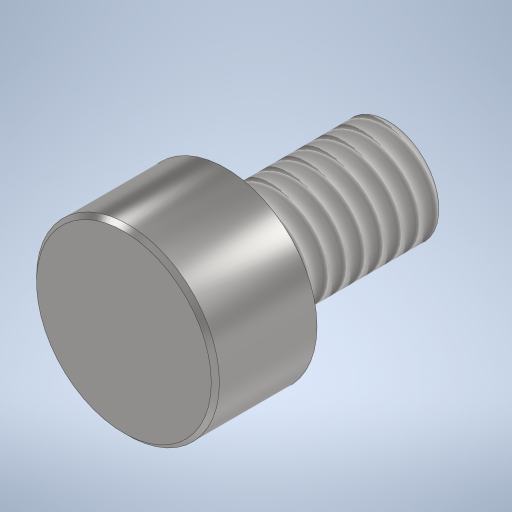
# Autodesk Inventor part: M2.5×4
Saved by Autodesk Inventor 2024 (Build 280153000, 153)
## iProperties
Created: 2025-03-04
Part Number: M2.5×4
Material: ステンレス鋼
Document SubType Name: Modeling
Designer: 1412z
Density: 8 g/cm^3
Appearance: 半つや出し
Author: 1412z
Autodesk Inventor part; units mm, degrees
ref_plane "YZ Plane" through (0, 0, 0) normal (1, 0, 0) x (0, 1, 0)
ref_plane "XZ Plane" through (0, 0, 0) normal (0, 1, 0) x (-1, 0, 0)
ref_plane "XY Plane" through (0, 0, 0) normal (0, 0, 1) x (1, 0, 0)
sketch "スケッチ1" plane through (0, 0, 0) normal (0, 0, 1) x (1, 0, 0)
  circle A0 centre (0, 0) radius 2.25
  dimension "d0" = 4.5
  constraints: 1 centre point, 1 coincident
  measures "d0" diameter of A0
extrude "押し出し1" add sketch "スケッチ1" along normal blind 2.5
sketch "スケッチ2" plane through (0, 0, 0) normal (0, 0, -1) x (-1, 0, 0)
  circle A0 centre (0, 0) radius 1.25
  dimension "d3" = 2.5
  constraints: 1 centre point, 1 coincident
  measures "d3" diameter of A0
extrude "押し出し2" add sketch "スケッチ2" along normal blind 4
chamfer "面取り1" distance 0.1 angle 45 1 edges at (-2.25, 0, 2.5)
thread "ねじ1" size "M2.5x0.45" class "6g" standard "ANSI Metric M Profile" full length
